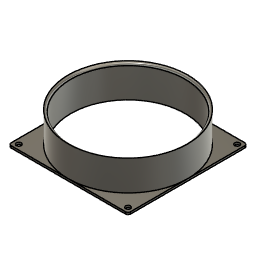
LianLiFanStab (Autodesk Fusion 360 design; units mm, degrees)
Autodesk Fusion 360 part; units mm, degrees
sketch "Sketch1" plane through (0, 0, 0) normal (0, 1, 0) x (1, 0, 0)
  line L0 (-106.5752, 68.8324) -> (8.4248, 68.8324)
  line L1 (10.9248, 66.3324) -> (10.9248, -48.6676)
  line L2 (8.4248, -51.1676) -> (-106.5752, -51.1676)
  line L3 (-109.0752, -48.6676) -> (-109.0752, 66.3324)
  line L4 (-49.0752, 68.8324) -> (-49.0752, -51.1676)
  line L5 (-109.0752, 8.8324) -> (10.9248, 8.8324)
  circle A0 centre (-49.0752, 8.8324) radius 57.5
  line L6 (-109.0752, 68.8324) -> (-103.9752, 68.8324)
  line L7 (-103.9752, 68.8324) -> (-103.9752, 63.7324)
  circle A1 centre (-103.9752, 63.7324) radius 2.5
  circle A2 centre (5.8248, 63.7324) radius 2.5
  circle A3 centre (-103.9752, -46.0676) radius 2.5
  circle A4 centre (5.8248, -46.0676) radius 2.5
  circle A5 centre (-49.0752, 8.8324) radius 60
  arc A6 (-109.0752, -48.6676) -> (-106.5752, -51.1676) centre (-106.5752, -48.6676) ccw
  arc A7 (8.4248, -51.1676) -> (10.9248, -48.6676) centre (8.4248, -48.6676) ccw
  arc A8 (10.9248, 66.3324) -> (8.4248, 68.8324) centre (8.4248, 66.3324) ccw
  arc A9 (-106.5752, 68.8324) -> (-109.0752, 66.3324) centre (-106.5752, 66.3324) ccw
  point P0 (10.9248, 68.8324)
  point P1 (10.9248, -51.1676)
  dimension "d1" = 120
  dimension "d2" = 120
  dimension "d3" = 115
  dimension "d4" = 5.1
  dimension "d6" = 5.1
  dimension "d7" = 5
  dimension "d8" = 2.5
  dimension "d9" = 2.5
  dimension "d10" = 2.5
  dimension "d11" = 2.5
  constraint horizontal L0
  constraint vertical L1
  constraint horizontal L2
  constraint vertical L3
  constraint midpoint L5 A0.centre
  constraint perpendicular L3 L6
  constraint perpendicular L6 L7
  constraint coincident L7.end A1.centre
  constraint symmetric L4 A1 A2
  constraint symmetric L5 A1 A3
  constraint symmetric L5 A2 A4
  constraint concentric A0 A5
  constraint coincident L5.start A5
  constraint coincident L3 L5.start
  constraint coincident L2 L4.end
  constraint tangent L3 A6
  constraint tangent L2 A6
  constraint coincident L1 L5.end
  constraint coincident P1 L2
  constraint coincident P1 L1
  constraint tangent L2 A7
  constraint tangent L1 A7
  constraint coincident L0 L4.start
  constraint coincident P0 L0
  constraint coincident P0 L1
  constraint tangent L0 A8
  constraint tangent L1 A8
  constraint coincident L6.start L0
  constraint coincident L6.start L3
  constraint tangent L0 A9
  constraint tangent L3 A9
  measures "d1" distance of L6.start P0
  measures "d2" distance of P0 P1
  measures "d3" diameter of A0
  measures "d4" distance of L6.start L6.end
  measures "d6" distance of L6.end L7.end
  measures "d7" diameter of A1
  measures "d8" radius of A6
  measures "d9" radius of A7
  measures "d10" radius of A8
  measures "d11" radius of A9
extrude "Extrude1" add sketch "Sketch1" along normal blind 2 contours L0 L3 L6 A5 A9 | L0 L1 A5 A8 | L2 L3 A5 A6 | L1 L2 A5 A7
extrude "Extrude2" add sketch "Sketch1" along normal blind 24 contours L4 L5 A0 A5 | L4 L5 A0 A5 | L4 L5 A0 A5 | L4 L5 A0 A5
fillet "Fillet1" radius 2 1 edges at (-102.684, 24, -29.6253)
extrude "Extrude3" add sketch "Sketch1" along normal blind 32.3 contours L4 L5 A0 A5 | L4 L5 A0 A5 | L4 L5 A0 A5 | L4 L5 A0 A5
fillet "Fillet2" radius 2.5 1 edges at (-102.684, 32.3, -29.6253)
